# Autodesk Inventor part: U_2_TILOGO_SMALL
Saved by Autodesk Inventor 2016 SP1 (Build 200210100, 210)
## iProperties
Created: 2015-11-24
Part Number: U_2_TILOGO_SMALL
Material: Generic
Document SubType Name: Modeling
Designer: PhillipD
Density: 1 g/cm^3
Appearance: TILOGO_SMALL, U_2_TILOGO_SMALL
Author: PhillipD
Autodesk Inventor part; units mm, degrees
ref_plane "YZ Plane" through (0, 0, 0) normal (1, 0, 0) x (0, 1, 0)
ref_plane "XZ Plane" through (0, 0, 0) normal (0, 1, 0) x (-1, 0, 0)
ref_plane "XY Plane" through (0, 0, 0) normal (0, 0, 1) x (1, 0, 0)
sketch "TILOGO_SMALL, U_2_TILOGO_SMALL_156" plane through (0, 0, 0) normal (0, 0, 1) x (1, 0, 0)
  line L0 (-1.2451, 0.7945) -> (0.9713, 0.7945)
  line L1 (0.9713, 0.7945) -> (0.9713, -1.3353)
  line L2 (0.9713, -1.3353) -> (-1.2451, -1.3353)
  line L3 (-1.2451, -1.3353) -> (-1.2451, 0.7945)
  constraints: 8 end point
extrude "Extrusion1" add sketch "TILOGO_SMALL, U_2_TILOGO_SMALL_156" along normal blind 1
body "Solid1"
